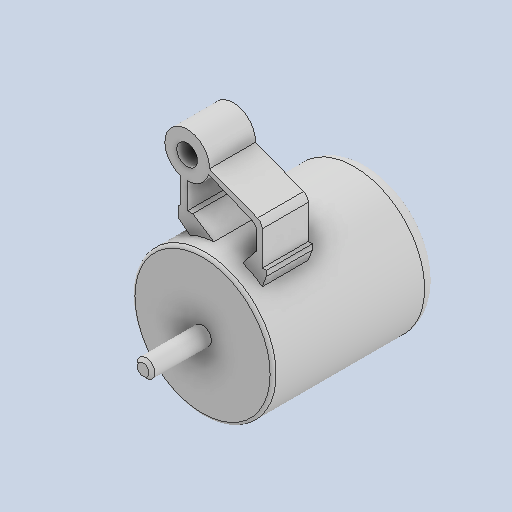
# Autodesk Inventor part: motor2
Saved by Autodesk Inventor 2022 (Build 260153000, 153)
## iProperties
Created: 2019-11-12
Part Number: motor2
Material: Genérico
Document SubType Name: Modeling
Designer: Usuario
Density: 1 g/cm^3
Appearance: Valor por defecto
Author: Usuario
Autodesk Inventor part; units mm, degrees
ref_plane "YZ Plane" through (0, 0, 0) normal (1, 0, 0) x (0, 1, 0)
ref_plane "XZ Plane" through (0, 0, 0) normal (0, 1, 0) x (-1, 0, 0)
ref_plane "XY Plane" through (0, 0, 0) normal (0, 0, 1) x (1, 0, 0)
sketch "Boceto1" plane through (0, 0, 0) normal (0, 0, 1) x (1, 0, 0)
  line L0 (0, 0) -> (176.0622, 0) construction
  line L1 (176.0622, 0) -> (176.0622, -234.7497) construction
  line L2 (176.0622, -234.7497) -> (0, -234.7497) construction
  line L3 (0, -234.7497) -> (0, 0) construction
  circle A0 centre (60.6994, -75.2554) radius 7
  line L4 (60.9494, -90.2533) -> (60.9494, -105.0535)
  line L5 (60.9494, -105.0535) -> (60.9494, -107.7044)
  line L6 (60.9494, -107.7044) -> (64.462, -107.7044)
  line L7 (64.462, -107.7044) -> (78.6909, -116.9211)
  arc A1 (62.497, -121.017) -> (111.2784, -126.8512) centre (82.0598, -164.3014) ccw
  line L8 (75.685, -75.9112) -> (111.2784, -89.6384)
  line L9 (111.2784, -89.6384) -> (111.2784, -91.0916)
  line L10 (111.2784, -91.0916) -> (111.2784, -115.9371)
  line L11 (111.2784, -115.9371) -> (114.0242, -115.9371)
  line L12 (114.0242, -115.9371) -> (114.0242, -119.5079)
  line L13 (114.0242, -119.5079) -> (111.2784, -126.8512)
  line L14 (75.0889, -79.491) -> (107.6439, -92.9034)
  line L15 (107.6439, -92.9034) -> (107.6439, -107.7044)
  line L16 (107.6439, -107.7044) -> (98.0464, -119.5725)
  line L17 (62.497, -121.017) -> (55.0669, -115.0084)
  line L18 (55.0669, -115.0084) -> (55.0669, -107.7044)
  line L19 (55.0669, -107.7044) -> (56.4416, -106.0045)
  line L20 (56.4416, -106.0045) -> (56.4416, -89.6384)
  arc A2 (75.0889, -79.491) -> (75.685, -75.9112) centre (60.6994, -75.2554) ccw construction
  arc A3 (60.9494, -90.2533) -> (75.0889, -79.491) centre (60.6994, -75.2554) ccw
  arc A4 (56.4416, -89.6384) -> (60.9494, -90.2533) centre (60.6994, -75.2554) ccw construction
  arc A5 (75.685, -75.9112) -> (56.4416, -89.6384) centre (60.6994, -75.2554) ccw
  arc A6 (78.6909, -116.9211) -> (62.497, -121.017) centre (82.0598, -164.3014) ccw construction
  arc A7 (111.2784, -126.8512) -> (98.0464, -119.5725) centre (82.0598, -164.3014) ccw construction
  arc A8 (98.0464, -119.5725) -> (78.6909, -116.9211) centre (82.0598, -164.3014) ccw
  dimension "d2" = 14
  dimension "d5" = 95
  dimension "d9" = 30
  constraints: 34 end point, 19 point on circle, 9 centre point, 5 perpendicular, 4 vertical, 3 point on line, 1 coincident, 1 parallel, 3 other
  measures "d2" diameter of A0
  measures "d5" diameter of A1
  measures "d9" diameter of A2
extrude "Extrusión1" add sketch "Boceto1" along normal blind 31
sketch "Boceto2" plane through (0, 0, 31) normal (0, 0, 1) x (1, 0, 0)
  arc A0 (62.497, -121.017) -> (111.2784, -126.8512) centre (82.0598, -164.3014) ccw projected
  circle A1 centre (82.0598, -164.3014) radius 47.5
  point P0 (0, 0)
  point P1 (62.497, -121.017)
  constraints: 1 coincident, 3 other
extrude "Extrusión2" add sketch "Boceto2" along normal blind 11
sketch "Boceto3" plane through (0, 0, 0) normal (0, 0, -1) x (-1, 0, 0)
  arc A0 (-111.2784, -126.8512) -> (-62.497, -121.017) centre (-82.0598, -164.3014) ccw projected
  circle A1 centre (-82.0598, -164.3014) radius 47.5
  point P0 (0, 0)
  constraints: 1 coincident, 3 other
extrude "Extrusión3" add sketch "Boceto3" along normal blind 70
fillet "Empalme1" radius 10 1 edges at (101.6226, -207.5859, -70)
fillet "Empalme2" radius 2 1 edges at (52.8411, -201.7517, 42)
sketch "Boceto4" plane through (82.0598, -164.3014, 42) normal (0, 0, 1) x (1, 0, 0)
  circle A0 centre (0, 0) radius 6
  point P0 (-82.0598, 164.3014)
  dimension "d32" = 12
  constraints: 1 centre point
  measures "d32" diameter of A0
extrude "Extrusión4" add sketch "Boceto4" along normal blind 40
chamfer "Chaflán1" distance 2 angle 45 1 edges at (76.0598, -164.3014, 82)
fillet "Empalme3" radius 5 2 edges at (111.2784, -89.6384, 15.5) (107.6439, -92.9034, 15.5)
